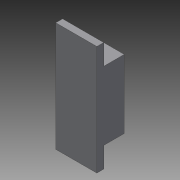
# Autodesk Inventor part: sonar
Saved by Autodesk Inventor 2015 SP1 (Build 190203100, 203)
## iProperties
Created: 2018-04-13
Part Number: sonar
Material: Generic
Document SubType Name: Modeling
Designer: 407642
Density: 1 g/cm^3
Appearance: Default
Author: 407642
Autodesk Inventor part; units mm, degrees
ref_plane "YZ Plane" through (0, 0, 0) normal (1, 0, 0) x (0, 1, 0)
ref_plane "XZ Plane" through (0, 0, 0) normal (0, 1, 0) x (-1, 0, 0)
ref_plane "XY Plane" through (0, 0, 0) normal (0, 0, 1) x (1, 0, 0)
sketch "Sketch1" plane through (0, 0, 0) normal (0, 1, 0) x (-1, 0, 0)
  line L0 (28.6465, 75.6443) -> (-1.3535, 75.6443)
  line L1 (-1.3535, 75.6443) -> (-1.3535, -4.3557)
  line L2 (-1.3535, -4.3557) -> (28.6465, -4.3557)
  line L3 (28.6465, -4.3557) -> (28.6465, 75.6443)
  point P0 (0, 0)
  dimension "d0" = 30
  dimension "d1" = 80
  constraints: 8 end point, 2 parallel, 1 horizontal, 1 perpendicular
  measures "d0" distance of L2.end L1.end
  measures "d1" distance of L1.end L0.end
extrude "Extrusion1" add sketch "Sketch1" along normal blind 5
sketch "Sketch2" plane through (0, 5, 0) normal (0, 1, 0) x (1, 0, 0)
  line L0 (1.3535, -75.6443) -> (1.3535, 4.3557) projected
  line L1 (-28.6465, -75.6443) -> (1.3535, -75.6443)
  line L2 (1.3535, -75.6443) -> (1.3535, -60.6443)
  line L3 (1.3535, -60.6443) -> (-28.6465, -60.6443)
  line L4 (-28.6465, -60.6443) -> (-28.6465, -75.6443)
  line L5 (-28.6465, 4.3557) -> (1.3535, 4.3557)
  line L6 (1.3535, 4.3557) -> (1.3535, -10.6443)
  line L7 (1.3535, -10.6443) -> (-28.6465, -10.6443)
  line L8 (-28.6465, -10.6443) -> (-28.6465, 4.3557)
  line L9 (-28.6465, -60.6443) -> (1.3535, -60.6443)
  line L10 (1.3535, -60.6443) -> (1.3535, -10.6443)
  line L11 (1.3535, -10.6443) -> (-28.6465, -10.6443)
  line L12 (-28.6465, -10.6443) -> (-28.6465, -60.6443)
  point P0 (0, 0)
  dimension "d4" = 15
  dimension "d5" = 15
  constraints: 24 end point, 6 parallel, 3 horizontal, 3 perpendicular, 2 point on line
  measures "d4" distance of L2.end L1.end
  measures "d5" distance of L5.end L6.end
extrude "Extrusion2" add sketch "Sketch2" along normal blind 15 contours L3 L12 L7 L0
sketch "Sketch3" plane through (0, 20, 0) normal (0, 1, 0) x (1, 0, 0)
  line L0 (1.3535, -60.6443) -> (-28.6465, -60.6443) projected
  line L1 (-13.6465, -60.6443) -> (-13.6465, -10.6443)
  line L2 (1.3535, -10.6443) -> (-28.6465, -10.6443) projected
  line L3 (-28.6465, 4.3557) -> (-28.6465, -75.6443) projected
  line L4 (-28.6465, -35.6443) -> (1.3535, -35.6443)
  line L5 (1.3535, -75.6443) -> (1.3535, 4.3557) projected
  line L6 (-13.6465, -60.6443) -> (-13.6465, -36.1443)
  line L7 (-13.6465, -60.6443) -> (-13.6465, -48.1443)
  circle A0 centre (-13.6465, -48.1443) radius 7.5
  circle A1 centre (-13.6465, -23.1443) radius 7.5
  point P0 (0, 0)
  dimension "d8" = 50
  dimension "d9" = 24.5
  dimension "d10" = 12.5
  dimension "d11" = 15
  constraints: 8 end point, 4 midpoint, 2 centre point, 2 point on line, 1 coincident, 1 symmetric about line, 1 other
  measures "d8" distance of L1.start L1.end
  measures "d9" distance of L1.start L6.end
  measures "d10" distance of L1.start L7.end
  measures "d11" diameter of A0
extrude "Extrusion4" cut sketch "Sketch3" against normal blind 8 contours A0 L1 | L1 A0 | A1 L1 | L1 A1
body "Solid1"
